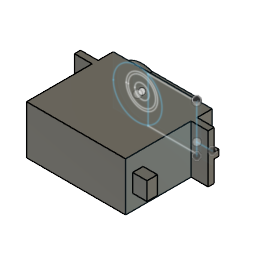
180 motor (Autodesk Fusion 360 design; units mm, degrees)
Autodesk Fusion 360 part; units mm, degrees
sketch "Sketch1" plane through (0, 0, 0) normal (0, 0, 1) x (1, 0, 0)
  line L0 (-20.375, 17.825) -> (20.375, 17.825)
  line L1 (20.375, 17.825) -> (20.375, -17.825)
  line L2 (20.375, -17.825) -> (-20.375, -17.825)
  line L3 (-20.375, -17.825) -> (-20.375, 17.825)
  line L4 (-20.375, 17.825) -> (20.375, -17.825) construction
  line L5 (20.375, 17.825) -> (-20.375, -17.825) construction
  dimension "d1" = 40.75
  dimension "d2" = 35.65
  constraint horizontal L0
  constraint perpendicular L0 L1
  constraint parallel L0 L2
  constraint parallel L1 L3
  constraint coincident L4 origin
  constraint coincident L5 origin
  measures "d1" distance of L1.end L2.end
  measures "d2" distance of L0.end L1.end
extrude "Extrude1" add sketch "Sketch1" along normal blind 20
sketch "Sketch2" plane through (20.375, 0, 0) normal (1, 0, 0) x (0, 1, 0)
  line L0 (-17.825, 0) -> (17.825, 0)
  line L1 (17.825, 0) -> (17.825, 20)
  line L2 (17.825, 20) -> (-17.825, 20)
  line L3 (-17.825, 20) -> (-17.825, 0)
  line L4 (17.825, 20) -> (11.625, 20)
  line L5 (11.625, 20) -> (9.125, 20)
  line L6 (9.125, 20) -> (9.125, 0)
  line L7 (9.125, 0) -> (11.625, 0)
  line L8 (11.625, 0) -> (11.625, 20)
  dimension "d5" = 6.2
  dimension "d6" = 2.5
  constraint coincident L1.end L2.start
  constraint perpendicular L1 L4
  constraint horizontal L5
  constraint vertical L6
  constraint horizontal L7
  constraint vertical L8
  constraint coincident L0 L6.end
  measures "d5" distance of L1.end L4.end
  measures "d6" distance of L4.end L5.end
extrude "Extrude2" add sketch "Sketch2" along normal blind 7 contours L0 L2 L5 L6 L7 L8
sketch "Sketch3" plane through (20.375, 0, 0) normal (1, 0, 0) x (0, 1, 0)
  line L0 (11.625, 20) -> (11.625, 0)
  line L1 (11.625, 0) -> (17.825, 0)
  line L2 (17.825, 0) -> (17.825, 20)
  line L3 (17.825, 20) -> (11.625, 20)
  line L4 (11.625, 20) -> (11.625, 11.25)
  line L5 (11.625, 0) -> (11.625, 8.75)
  line L6 (17.825, 10) -> (13.575, 10)
  line L7 (11.625, 11.25) -> (13.575, 11.25)
  line L8 (13.575, 11.25) -> (13.575, 10)
  line L9 (13.575, 10) -> (11.625, 10)
  line L10 (11.625, 10) -> (11.625, 11.25)
  line L11 (13.575, 10) -> (11.625, 10)
  line L12 (11.625, 10) -> (11.625, 8.75)
  line L13 (11.625, 8.75) -> (13.575, 8.75)
  line L14 (13.575, 8.75) -> (13.575, 10)
  dimension "d9" = 8.75
  dimension "d10" = 8.75
  dimension "d11" = 4.25
  constraint coincident L0.start L3.end
  constraint perpendicular L3 L4
  constraint coincident L0.end L1.start
  constraint perpendicular L1 L5
  constraint midpoint L2 L6.start
  constraint perpendicular L0 L6
  constraint horizontal L7
  constraint vertical L8
  constraint horizontal L9
  constraint vertical L10
  constraint horizontal L11
  constraint vertical L12
  constraint horizontal L13
  constraint vertical L14
  measures "d9" distance of L0.start L4.end
  measures "d10" distance of L0.end L5.end
  measures "d11" distance of L6.start L6.end
extrude "Extrude3" add sketch "Sketch3" along normal blind 7 contours L0 L7 L8 L9 L10 L11 | L0 L9 L11 L12 L13 L14
extrude "Extrude4" add 1 faces at (27.375, 9.9583, 9.5833) along direction (-1, 0, 0) blind 55
sketch "Sketch4" plane through (20.375, 0, 0) normal (1, 0, 0) x (0, 1, 0)
  line L0 (9.125, 0) -> (9.125, 20)
  line L1 (9.125, 20) -> (-17.825, 20)
  line L2 (-17.825, 20) -> (-17.825, 0)
  line L3 (-17.825, 0) -> (9.125, 0)
sketch "Sketch5" plane through (20.375, 0, 0) normal (1, 0, 0) x (0, 1, 0)
  line L0 (-15, 20) -> (-15, 13.7)
  line L1 (-17.8217, 13.7) -> (-14.9217, 13.7)
  line L2 (-14.9217, 0) -> (-14.9217, 6.3)
  line L3 (-14.9217, 6.3) -> (-10.6217, 6.3)
  line L4 (-10.6217, 6.3) -> (-10.6217, 13.7)
  line L5 (-10.6217, 13.7) -> (-14.9217, 13.7)
  line L6 (-14.9217, 13.7) -> (-14.9217, 6.3)
  dimension "d16" = 6.3
  dimension "d17" = 2.9
  dimension "d18" = 6.3
  dimension "d19" = 4.3
  constraint vertical L0
  constraint perpendicular L0 L1
  constraint perpendicular L1 L2
  constraint horizontal L3
  constraint vertical L4
  constraint horizontal L5
  constraint vertical L6
  measures "d16" distance of L0.start L0.end
  measures "d17" distance of L1.start L1.end
  measures "d18" distance of L2.start L2.end
  measures "d19" distance of L2.end L3.end
extrude "Extrude5" add sketch "Sketch5" along normal blind 5.9
sketch "Sketch6" plane through (0, 17.825, 0) normal (0, 1, 0) x (-1, 0, 0)
  line L0 (-20.375, 0) -> (20.375, 0)
  line L1 (20.375, 0) -> (20.375, 20)
  line L2 (20.375, 20) -> (-20.375, 20)
  line L3 (-20.375, 20) -> (-20.375, 0)
  line L4 (-20.375, 4.9972) -> (-14.025, 4.9972)
  line L5 (-14, 0) -> (-14, 0.75)
  line L6 (-14, 20) -> (-14, 19.25)
  line L7 (-14, 0.75) -> (6, 0.75)
  line L8 (6, 0.75) -> (6, 19.25)
  line L9 (6, 19.25) -> (-14, 19.25)
  line L10 (-14, 19.25) -> (-14, 0.75)
  circle A0 centre (10.3, 10) radius 10
  dimension "d22" = 6.35
  dimension "d23" = 0.75
  dimension "d24" = 0.75
  dimension "d25" = 20
  dimension "d26" = 18.5
  constraint coincident L3 L4.start
  constraint perpendicular L3 L4
  constraint coincident L0 L5.start
  constraint perpendicular L0 L5
  constraint coincident L2 L6.start
  constraint perpendicular L2 L6
  constraint horizontal L7
  constraint vertical L8
  constraint horizontal L9
  constraint vertical L10
  measures "d22" distance of L4.start L4.end
  measures "d23" distance of L5.start L5.end
  measures "d24" distance of L6.start L6.end
  measures "d25" distance of L5.end L7.end
  measures "d26" distance of L5.end L6.end
extrude "Extrude6" add sketch "Sketch6" along normal blind 1.75 contours L8 A0 | L7 L8 L9 L10 A0 | L8 A0
sketch "Sketch7" plane through (0, 19.575, 0) normal (0, 1, 0) x (-1, 0, 0)
  arc A0 (6, 0.9717) -> (6, 19.0283) centre (10.3, 10) ccw
  line L0 (6, 19.0283) -> (6, 19.25)
  line L1 (6, 19.25) -> (-14, 19.25)
  line L2 (-14, 19.25) -> (-14, 0.75)
  line L3 (-14, 0.75) -> (6, 0.75)
  line L4 (6, 0.75) -> (6, 0.9717)
  circle A1 centre (10.3, 10) radius 6.45
  circle A2 centre (10.3, 10) radius 5.6
  circle A3 centre (10.3, 10) radius 2.9
  dimension "d29" = 12.9
  dimension "d30" = 11.2
  dimension "d31" = 5.8
  constraint concentric A0 A1
  constraint concentric A1 A2
  constraint concentric A1 A3
  measures "d29" diameter of A1
  measures "d30" diameter of A2
  measures "d31" diameter of A3
extrude "Extrude7" add sketch "Sketch7" along normal blind 1.4 contours A1
extrude "Extrude8" add 1 faces at (-12.8422, 19.575, 11.496) along direction (0, 1, 0) blind 2.1
sketch "Sketch8" plane through (0, 21.675, 0) normal (0, 1, 0) x (-1, 0, 0)
  circle A0 centre (10.3, 10) radius 5.6
sketch "Sketch9" plane through (0, 21.675, 0) normal (0, 1, 0) x (-1, 0, 0)
  circle A0 through (13.2, 10, -2.1) (8.85, 12.5115, -2.1) (8.85, 7.4885, -2.1)
  circle A1 centre (10.3, 10) radius 2.9063
  circle A2 centre (10.3, 10) radius 5.6
  circle A3 centre (10.3, 10) radius 2.9063
  point P0 (10.3, 10)
  constraint coincident P0 A1.centre
  constraint concentric A1 A2
  constraint concentric A1 A3
extrude "Extrude9" add sketch "Sketch9" along normal blind 3.5 contours A1 A3
sketch "Sketch10" plane through (0, 17.825, 0) normal (0, 1, 0) x (-1, 0, 0)
  arc A0 (10.3, 20) -> (6, 19.0283) centre (10.3, 10) ccw
  line L0 (10.3, 20) -> (-20.375, 20)
  line L1 (-20.375, 20) -> (-20.375, 0)
  line L2 (-20.375, 0) -> (10.3, 0)
  arc A1 (6, 0.9717) -> (10.3, 0) centre (10.3, 10) ccw
  line L3 (6, 0.9717) -> (6, 0.75)
  line L4 (6, 0.75) -> (-14, 0.75)
  line L5 (-14, 0.75) -> (-14, 19.25)
  line L6 (-14, 19.25) -> (6, 19.25)
  line L7 (6, 19.25) -> (6, 19.0283)
  line L8 (-14, 14.875) -> (-14, 5.125)
  circle A2 centre (-12.2062, 10.0187) radius 5.0718
  point P0 (-14, 10)
  dimension "d38" = 9.75
  constraint midpoint L8 P0
  constraint coincident L5 P0
  constraint perpendicular L4 L8
  measures "d38" distance of L8.start L8.end
extrude "Extrude10" add sketch "Sketch10" along normal blind 1.75 contours L5 L8 A2 picked at (-15.8122, 10.2321)
